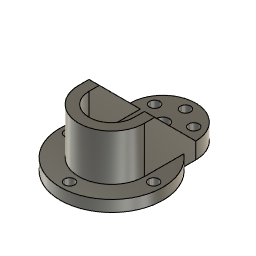
NCV-09 v1 (Autodesk Fusion 360 design; units mm, degrees)
Autodesk Fusion 360 part; units mm, degrees
sketch "Sketch1" plane through (0, 0, 0) normal (0, 0, 1) x (1, 0, 0)
  circle A0 centre (-41, 0) radius 5
  line L0 (-32, 50) -> (-32, 0)
  line L1 (32, 50) -> (32, 0)
  arc A1 (-32, 38.4187) -> (32, 38.4187) centre (0, 0) ccw
  arc A2 (-32, 25.632) -> (32, 25.632) centre (0, 0) ccw construction
  arc A3 (-32, 0) -> (32, 0) centre (0, 0) ccw
  arc A4 (32, 50) -> (-32, 50) centre (0, 50) ccw
  circle A5 centre (0, 50) radius 22 construction
  circle A6 centre (0, 72) radius 5
  line L2 (6, 50) -> (6, 0)
  line L3 (-6, 50) -> (-6, 0)
  arc A7 (-6, 0) -> (6, 0) centre (0, 0) ccw
  arc A8 (6, 50) -> (-6, 50) centre (0, 50) ccw
  line L4 (-32, 50) -> (-22, 50)
  line L5 (32, 50) -> (22, 50)
  line L6 (-22, 50) -> (-22, 0)
  line L7 (22, 50) -> (22, 0)
  arc A9 (-22, 0) -> (22, 0) centre (0, 0) ccw
  line L8 (-32, 12) -> (-22, 12)
  line L9 (22, 12) -> (32, 12)
  dimension "d1" = 100
  dimension "d2" = 82
  dimension "d3" = 10
  dimension "d4" = 41
  dimension "d5" = 64
  dimension "d6" = 64
  dimension "d7" = 50
  dimension "d8" = 50
  dimension "d9" = 12
  dimension "d10" = 12
  dimension "d11" = 44
  dimension "d12" = 44
  dimension "d13" = 10
  dimension "d14" = 22
  dimension "d15" = 12
  dimension "d16" = 12
  constraint coincident A1.centre A2.centre
  constraint coincident A0.centre A2
  constraint concentric A1 A3
  constraint vertical L1
  constraint vertical L0
  constraint tangent L0 A3
  constraint tangent L1 A3
  constraint tangent L1 A4
  constraint coincident L0 A1.start
  constraint coincident L1 A1.end
  constraint coincident L1 A2.end
  constraint coincident L0 A2.start
  constraint concentric A4 A8
  constraint concentric A3 A7
  constraint concentric A5 A8
  constraint concentric A1 A9
  constraint coincident A5 A6.centre
  constraint vertical L3
  constraint vertical L2
  constraint tangent L3 A8
  constraint tangent L2 A8
  constraint coincident A5 L4.end
  constraint coincident A5 L5.end
  constraint horizontal L4
  constraint horizontal L5
  constraint vertical L6
  constraint vertical L7
  constraint coincident L0 L8.start
  constraint coincident L6 L8.end
  constraint coincident L7 L9.start
  constraint coincident L1 L9.end
  constraint horizontal L8
  constraint horizontal L9
  measures "d1" diameter of A1
  measures "d2" diameter of A2
  measures "d3" diameter of A0
  measures "d4" horizontal distance of A1.centre A0.centre
  measures "d5" diameter of A3
  measures "d6" diameter of A4
  measures "d7" vertical distance of A1.centre A4.centre
  measures "d8" vertical distance of A1.centre L0.start
  measures "d9" diameter of A8
  measures "d10" diameter of A7
  measures "d11" diameter of A5
  measures "d12" diameter of A9
  measures "d13" diameter of A6
  measures "d14" vertical distance of A4.centre A6.centre
  measures "d15" distance of A1.centre L9
  measures "d16" distance of A1.centre L8
extrude "Extrude1" add sketch "Sketch1" against normal blind 16 contours A0 | L0 L1 A1 A3 makes body 1
extrude "Extrude3" cut sketch "Sketch1" against normal blind 5 contours A0 | L0 L1 A1 A3 bodies 1
extrude "Extrude2" add sketch "Sketch1" against normal blind 16 separate body contours A4 L4 L5 L6 L7 A9 | A6 makes body 2
extrude "Extrude4" add sketch "Sketch1" along normal blind 40 and the other way up to surface (16 mm away) contours L0 L4 L6 L8 | L1 L5 L7 L9 | L0 L1 A3 L6 L7 A9 L8 L9 bodies 1 2
chamfer "Chamfer1" distance 40 angle 45 2 edges at (-27, 50, 40) (27, 50, 40) on bodies 1
extrude "Extrude6" cut sketch "Sketch1" against normal through all contours A0 bodies 1
extrude "Extrude7" cut sketch "Sketch1" against normal through all contours A6 bodies 1
pattern_circular "C-Pattern1" count 3 over 180 about axis through (0, 0, 1.75) along (0, 0, 1) of "Extrude6"
pattern_circular "C-Pattern2" count 3 over 120 about axis through (0, 50, 0) along (0, 0, -1) both ways of "Extrude7"
equation "d4 = d2 / 2"
equation "d14 = d11 / 2"
